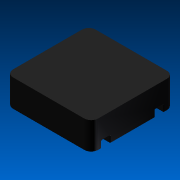
# Autodesk Inventor part: 12mm Incremental Encoder Base
Saved by Autodesk Inventor 2014 (Build 180170000, 170)
## iProperties
Created: 2011-11-07
Part Number: 12mm Incremental Encoder Base
Document SubType Name: Modeling
Designer: sdarley
Density: 1 g/cm^3
Material: Generic
Appearance: Glossy - Black
Author: sdarley
Autodesk Inventor part; units mm, degrees
ref_plane "YZ Plane" through (0, 0, 0) normal (1, 0, 0) x (0, 1, 0)
ref_plane "XZ Plane" through (0, 0, 0) normal (0, 1, 0) x (-1, 0, 0)
ref_plane "XY Plane" through (0, 0, 0) normal (0, 0, 1) x (1, 0, 0)
sketch "Sketch1" plane through (0, 0, 0) normal (0, 0, 1) x (1, 0, 0)
  line L0 (-5.175, 6) -> (5.175, 6)
  line L1 (6.175, 5) -> (6.175, -5)
  line L2 (5.175, -6) -> (-5.175, -6)
  line L3 (-6.175, -5) -> (-6.175, 5)
  arc A0 (-5.175, 6) -> (-6.175, 5) centre (-5.175, 5) ccw
  arc A1 (6.175, 5) -> (5.175, 6) centre (5.175, 5) ccw
  arc A2 (-6.175, -5) -> (-5.175, -6) centre (-5.175, -5) ccw
  arc A3 (5.175, -6) -> (6.175, -5) centre (5.175, -5) ccw
  point P0 (0, 0)
  point P1 (0, 6)
  point P2 (-6.175, 0)
  dimension "d0" = 12.35
  dimension "d1" = 12
  dimension "d2" = 1
  constraints: 8 end point, 8 point on circle, 8 tangent, 4 centre point, 3 equal radius, 2 midpoint, 2 parallel, 1 horizontal, 1 horizontal alignment, 1 perpendicular, 1 vertical alignment
  measures "d0" distance between parallel lines of L1 L3
  measures "d1" distance between parallel lines of L2 L0
  measures "d2" radius of A0
extrude "Extrusion1" add sketch "Sketch1" along normal blind 4
sketch "Sketch2" plane through (6.175, -5, 0) normal (1, 0, 0) x (0, 0, -1)
  line L0 (0, 10) -> (0, 0) projected
  line L1 (0, 9.5) -> (-1, 9.5)
  line L2 (-1, 9.5) -> (-1, 8.25)
  line L3 (-1, 8.25) -> (0, 8.25)
  line L4 (0, 8.25) -> (0, 9.5)
  line L5 (0, 0.5) -> (-1, 0.5)
  line L6 (-1, 0.5) -> (-1, 1.75)
  line L7 (-1, 1.75) -> (0, 1.75)
  line L8 (0, 1.75) -> (0, 0.5)
  point P0 (0, 5)
  dimension "d5" = 1.25
  dimension "d6" = 1.25
  dimension "d11" = 1
  dimension "d12" = 1
  constraints: 16 end point, 4 parallel, 2 horizontal, 2 perpendicular, 2 point on line
  measures "d5" distance of L2.end L1.end
  measures "d6" distance of L5.end L6.end
  measures "d11" distance between parallel lines of L0 L2
  measures "d12" distance between parallel lines of L0 L6
extrude "Extrusion2" cut sketch "Sketch2" against normal through all
fillet "Fillet1" radius 0.1 8 edges at (0, -4.5, 0) (0, -4.5, 1) (0, -3.25, 1) (0, -3.25, 0) (0, 3.25, 1) (0, 4.5, 1) (0, 4.5, 0) (0, 3.25, 0)
fillet "Fillet2" radius 0.1 40 edges at (6.175, 0, 0) (6.175, -3.2207, 0.0293) (6.175, -3.25, 0.5) (6.175, -3.2793, 0.9707) (6.175, -3.875, 1) (6.175, -4.4707, 0.9707) (6.175, -4.5, 0.5) (6.175, -4.5293, 0.0293) (6.175, -4.8, 0) (5.8821, -5.7071, 0) (0, -6, 0) (-5.8821, -5.7071, 0) (-6.175, -4.8, 0) (-6.175, -4.5293, 0.0293) (-6.175, -4.5, 0.5) (-6.175, -4.4707, 0.9707) (-6.175, -3.875, 1) (-6.175, -3.2793, 0.9707) (-6.175, -3.25, 0.5) (-6.175, -3.2207, 0.0293) (-6.175, 0, 0) (-6.175, 3.2207, 0.0293) (-6.175, 3.25, 0.5) (-6.175, 3.2793, 0.9707) (-6.175, 3.875, 1) (-6.175, 4.4707, 0.9707) (-6.175, 4.5, 0.5) (-6.175, 4.5293, 0.0293) (-6.175, 4.8, 0) (-5.8821, 5.7071, 0) (0, 6, 0) (5.8821, 5.7071, 0) (6.175, 4.8, 0) (6.175, 4.5293, 0.0293) (6.175, 4.5, 0.5) (6.175, 4.4707, 0.9707) (6.175, 3.875, 1) (6.175, 3.2793, 0.9707) (6.175, 3.25, 0.5) (6.175, 3.2207, 0.0293)
equation "\"d6\" = d5"
equation "\"d12\" = d11"
body "Solid1"
